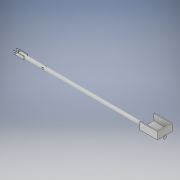
# Autodesk Inventor part: PBotArm
Saved by Autodesk Inventor 2018 (Build 220112000, 112)
## iProperties
Created: 2018-05-31
Part Number: PBotArm
Material: Generic
Document SubType Name: Modeling
Designer: choices
Density: 1 g/cm^3
Appearance: Default
Author: choices
Autodesk Inventor part; units mm, degrees
ref_plane "YZ Plane" through (0, 0, 0) normal (1, 0, 0) x (0, 1, 0)
sketch "Sketch1" plane through (0, 0, 0) normal (1, 0, 0) x (0, 1, 0)
  circle A0 centre (0, 0) radius 10.7315
  dimension "d0" = 21.463
  constraints: 1 centre point, 1 coincident
  measures "d0" diameter of A0
extrude "Extrusion1" add sketch "Sketch1" along normal blind 1047.75
sketch "Sketch2" plane through (1047.75, 0, 0) normal (1, 0, 0) x (0, 0, -1)
  circle A0 centre (0, 0) radius 10.7315 projected
  circle A1 centre (0, 0) radius 10.7315 projected
  line L0 (0, 10.7315) -> (53.975, 10.7315)
  line L1 (53.975, 10.7315) -> (53.975, 61.5315)
  line L2 (53.975, 61.5315) -> (0, 61.5315)
  line L3 (0, 10.7315) -> (-53.975, 10.7315)
  line L4 (-53.975, 10.7315) -> (-53.975, 61.5315)
  line L5 (-53.975, 61.5315) -> (0, 61.5315)
  circle A2 centre (0, 0) radius 10.7315 projected
  line L6 (-53.975, 61.5315) -> (53.975, 61.5315)
  line L7 (53.975, 61.5315) -> (53.975, 10.7315)
  line L8 (53.975, 10.7315) -> (-53.975, 10.7315)
  line L9 (-53.975, 10.7315) -> (-53.975, 61.5315)
  dimension "d5" = 107.95
  dimension "d6" = 50.8
  constraints: 20 end point, 4 horizontal, 4 parallel, 3 perpendicular, 2 vertical alignment, 1 point on line, 1 other
  measures "d5" distance between parallel lines of L4 L1
  measures "d6" distance of L3.end L4.end
extrude "Extrusion2" add sketch "Sketch2" against normal blind 127 contours L3 L4 L5 L2 L1 L0
shell "Shell1" thickness 6.35 removed faces 1 at (1005.4167, 61.5315, -17.9917)
sketch "Sketch3" plane through (927.1, 17.0815, -47.625) normal (1, 0, 0) x (0, 0, -1)
  line L0 (0, 44.45) -> (0, 0) projected
  line L1 (-95.25, 44.45) -> (0, 44.45) projected
  line L2 (-95.25, 0) -> (-95.25, 44.45) projected
  line L3 (0, 0) -> (-95.25, 0) projected
  point P0 (-47.625, -17.0815)
extrude "Extrusion3" cut sketch "Sketch3" against normal blind 127
sketch "Sketch4" plane through (1047.75, 10.7315, 53.975) normal (0, 0, 1) x (1, 0, 0)
  line L0 (-1041.4, -6.35) -> (-6.35, -6.35) projected
  line L1 (-1047.75, 0) -> (0, 0) projected
  line L2 (-1047.75, -21.463) -> (0, -21.463) projected
  line L3 (-1047.75, 0) -> (-1047.75, -21.463) projected
  line L4 (0, -21.463) -> (0, 0) projected
  circle A0 centre (-1027.7374, -10.7315) radius 6.35
  circle A1 centre (-869.95, -10.7315) radius 6.35
  point P0 (-1047.75, -10.7315)
  dimension "d12" = 12.7
  dimension "d13" = 12.7
  dimension "d14" = 869.95
  constraints: 2 centre point
  measures "d12" diameter of A0
  measures "d13" diameter of A1
  measures "d14" distance from line of L4 A1.centre
extrude "Extrusion4" cut sketch "Sketch4" against normal blind 127 contours A1 L0 | L0 A1
ref_plane "Work Plane1" through (0, 0, -10.7315) normal (0, 0, 1) x (1, 0, 0)
sketch "Sketch6" plane through (0, 0, -10.7315) normal (0, 0, 1) x (1, 0, 0)
  line L0 (0, 10.7315) -> (1047.75, 10.7315) projected
  line L1 (0, 10.7315) -> (0, -10.7315) projected
  line L2 (0, -10.7315) -> (1047.75, -10.7315) projected
  line L3 (-31.75, 10.7315) -> (44.45, 10.7315)
  line L4 (44.45, 10.7315) -> (44.45, -10.7315)
  line L5 (44.45, -10.7315) -> (-31.75, -10.7315)
  line L6 (-31.75, -10.7315) -> (-31.75, 10.7315)
  point P0 (0, 0)
  dimension "d18" = 76.2
  dimension "d19" = 44.45
  constraints: 8 end point, 2 parallel, 1 collinear, 1 horizontal, 1 perpendicular, 1 point on line
  measures "d18" distance of L4.end L5.end
  measures "d19" distance between parallel lines of L4 L1
extrude "Extrusion5" add sketch "Sketch6" against normal blind 3.175
ref_plane "Work Plane2" through (0, 0, 10.7315) normal (0, 0, 1) x (1, 0, 0)
sketch "Sketch7" plane through (0, 0, 10.7315) normal (0, 0, 1) x (1, 0, 0)
  line L0 (44.45, -10.7315) -> (44.45, 0) projected
  line L1 (0, 0) -> (44.45, 0) projected
  line L2 (44.45, 0) -> (44.45, 10.7315) projected
  line L3 (44.45, 10.7315) -> (-31.75, 10.7315) projected
  line L4 (-31.75, 10.7315) -> (-31.75, -10.7315) projected
  line L5 (-31.75, -10.7315) -> (44.45, -10.7315) projected
extrude "Extrusion6" add sketch "Sketch7" along normal blind 3.175
sketch "Sketch8" plane through (0, 0, -13.9065) normal (0, 0, -1) x (-1, 0, 0)
  circle A0 centre (16.51, 0) radius 6.35
  line L0 (31.75, -10.7315) -> (31.75, 10.7315) projected
  point P0 (0, 0)
  dimension "d24" = 12.7
  dimension "d25" = 15.24
  constraints: 1 centre point
  measures "d24" diameter of A0
  measures "d25" distance from line of L0 A0.centre
extrude "Extrusion7" cut sketch "Sketch8" against normal up to surface (27.813 mm away)
body "Solid1"
